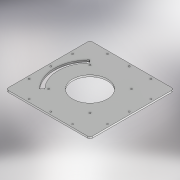
# Autodesk Inventor part: BaseTopPlate
Saved by Autodesk Inventor 2020.3 (Build 243373000, 373)
## iProperties
Created: 2021-08-02
Part Number: BaseTopPlate
Material: Aluminum
Document SubType Name: Modeling
Designer: justi
Density: 2.7 g/cm^3
Appearance: Aluminum - Polished
Author: justi
Autodesk Inventor part; units mm, degrees
ref_plane "YZ Plane" through (0, 0, 0) normal (1, 0, 0) x (0, 1, 0)
ref_plane "XZ Plane" through (0, 0, 0) normal (0, 1, 0) x (-1, 0, 0)
ref_plane "XY Plane" through (0, 0, 0) normal (0, 0, 1) x (1, 0, 0)
sketch "Sketch1" plane through (0, 0, 0) normal (0, 1, 0) x (-1, 0, 0)
  line L0 (-145, -145) -> (145, -145)
  line L1 (145, -145) -> (145, 145)
  line L2 (145, 145) -> (-145, 145)
  line L3 (-145, 145) -> (-145, -145)
  line L4 (-145, -145) -> (145, 145) construction
  line L5 (145, -145) -> (-145, 145) construction
  circle A0 centre (0, 0) radius 60
  line L6 (135, 135) -> (135, -135) construction
  line L7 (135, -135) -> (-135, -135) construction
  line L8 (-135, -135) -> (-135, 135) construction
  line L9 (-135, 135) -> (135, 135) construction
  line L10 (145, 135) -> (125, 135) construction
  line L11 (125, 135) -> (125, -135) construction
  line L12 (-145, 135) -> (-125, 135) construction
  line L13 (-125, 135) -> (-125, -135) construction
  line L14 (-125, 135) -> (125, 135) construction
  line L15 (-125, -135) -> (125, -135) construction
  line L16 (135, 125) -> (135, -125) construction
  line L17 (-135, 125) -> (-135, -125) construction
  circle A1 centre (0, -135) radius 2.75
  line L18 (0, -135) -> (75, -135)
  line L19 (0, -135) -> (-75, -135)
  circle A2 centre (75, -135) radius 2.75
  circle A3 centre (-75, -135) radius 2.75
  line L20 (0, 135) -> (75, 135)
  line L21 (0, 135) -> (-75, 135)
  circle A4 centre (75, 135) radius 2.75
  circle A5 centre (0, 135) radius 2.75
  circle A6 centre (-75, 135) radius 2.75
  line L22 (135, 0) -> (135, -75)
  line L23 (135, 0) -> (135, 75)
  circle A7 centre (135, -75) radius 2.75
  circle A8 centre (135, 0) radius 2.75
  circle A9 centre (135, 75) radius 2.75
  line L24 (-135, 0) -> (-135, -75)
  line L25 (-135, 0) -> (-135, 75)
  circle A10 centre (-135, -75) radius 2.75
  circle A11 centre (-135, 0) radius 2.75
  circle A12 centre (-135, 75) radius 2.75
  dimension "d0" = 290
  dimension "d1" = 290
  dimension "d2" = 120
  dimension "d3" = 10
  dimension "d4" = 20
  dimension "d5" = 20
  dimension "d29" = 5.5
  dimension "d30" = 75
  dimension "d31" = 75
  dimension "d32" = 5.5
  dimension "d33" = 5.5
  dimension "d34" = 75
  dimension "d35" = 75
  dimension "d36" = 5.5
  dimension "d37" = 5.5
  dimension "d38" = 5.5
  dimension "d39" = 75
  dimension "d40" = 75
  dimension "d41" = 5.5
  dimension "d42" = 5.5
  dimension "d43" = 5.5
  dimension "d44" = 75
  dimension "d45" = 75
  dimension "d46" = 5.5
  dimension "d47" = 5.5
  dimension "d48" = 5.5
  constraints: 60 end point, 17 point on line, 13 centre point, 13 coincident, 10 midpoint, 4 parallel, 4 perpendicular, 2 collinear, 1 horizontal, 3 other
  measures "d0" distance of L2.end L1.end
  measures "d1" distance of L1.end L0.end
  measures "d2" diameter of A0
  measures "d3" distance between parallel lines of L1 L6
  measures "d4" distance of L10.start L10.end
  measures "d5" distance of L12.start L12.end
  measures "d29" diameter of A1
  measures "d30" distance of L18.start L18.end
  measures "d31" distance of L18.start L19.end
  measures "d32" diameter of A2
  measures "d33" diameter of A3
  measures "d34" distance of L20.start L20.end
  measures "d35" distance of L20.start L21.end
  measures "d36" diameter of A4
  measures "d37" diameter of A5
  measures "d38" diameter of A6
  measures "d39" distance of L22.start L22.end
  measures "d40" distance of L22.start L23.end
  measures "d41" diameter of A7
  measures "d42" diameter of A8
  measures "d43" diameter of A9
  measures "d44" distance of L24.start L24.end
  measures "d45" distance of L24.start L25.end
  measures "d46" diameter of A10
  measures "d47" diameter of A11
  measures "d48" diameter of A12
extrude "Extrusion1" add sketch "Sketch1" against normal blind 6 contours L3 L2 L1 L0 | L18 L19 A1 | A1 L19 L18 | A2 | A3 | L21 A5 L20 | L20 A5 L21 | A4 | A6 | L23 A8 L22 | L22 A8 L23 | A7 | A9 | L25 A11 L24 | L24 A11 L25 | A10 | A12
fillet "Fillet1" radius 8 4 edges at (-145, -3, -145) (-145, -3, 145) (145, -3, 145) (145, -3, -145)
extrude "Extrusion2" cut sketch "Sketch1" against normal through all contours L18 L19 A1 | A1 L19 L18 | A2 | A3 | L21 A5 L20 | L20 A5 L21 | A4 | A6 | L23 A8 L22 | L22 A8 L23 | A7 | A9 | L25 A11 L24 | L24 A11 L25 | A10 | A12
sketch "Sketch3" plane through (0, 0, 0) normal (0, 1, 0) x (1, 0, 0)
  line L0 (-71.5, 71.5) -> (71.5, 71.5)
  line L1 (71.5, 71.5) -> (71.5, -71.5)
  line L2 (71.5, -71.5) -> (-71.5, -71.5)
  line L3 (-71.5, -71.5) -> (-71.5, 71.5)
  line L4 (-71.5, 71.5) -> (71.5, -71.5) construction
  line L5 (71.5, 71.5) -> (-71.5, -71.5) construction
  point P0 (0, 0)
  dimension "d51" = 143
  dimension "d52" = 143
  constraints: 12 end point, 2 midpoint, 2 parallel, 1 horizontal, 1 perpendicular
  measures "d51" distance of L1.end L2.end
  measures "d52" distance of L0.end L1.end
hole "Hole2" at (-71.5, 0, 71.5) at (-71.5, 0, -71.5) at (71.5, 0, -71.5) at (71.5, 0, 71.5) direction (0, -1, 0) diameter 5.5 end through all
sketch "Sketch4" plane through (0, 0, 0) normal (0, 1, 0) x (1, 0, 0)
  line L0 (0, 0) -> (-110, 0) construction
  line L1 (-145, 137) -> (-145, -137) projected
  arc A0 (-77.7817, 77.7817) -> (-77.7817, -77.7817) centre (0, 0) ccw
  arc A1 (-86.9199, 86.9199) -> (-86.9199, -86.9199) centre (0, 0) ccw
  line L2 (-77.7817, 77.7817) -> (-86.9199, 86.9199)
  line L3 (0, 0) -> (222.1817, 0) construction
  line L4 (-77.7817, -77.7817) -> (-86.9199, -86.9199)
  line L5 (0, 0) -> (151.3127, 0) construction
  dimension "d60" = 110
  dimension "d61" = 135
  dimension "d62" = 135
  constraints: 10 end point, 5 point on circle, 2 centre point, 2 coincident, 2 horizontal, 1 perpendicular
  measures "d60" distance of L0.start L0.end
  measures "d61" angle of L3 L2
  measures "d62" angle of L4 L5
extrude "Extrusion3" cut sketch "Sketch4" against normal blind 10
fillet "Fillet2" radius 2 4 edges at (-77.7817, -3, -77.7817) (-86.9199, -3, -86.9199) (-86.9199, -3, 86.9199) (-77.7817, -3, 77.7817)
equation "\"d32\" = d29"
equation "\"d33\" = d29"
body "Solid1"
